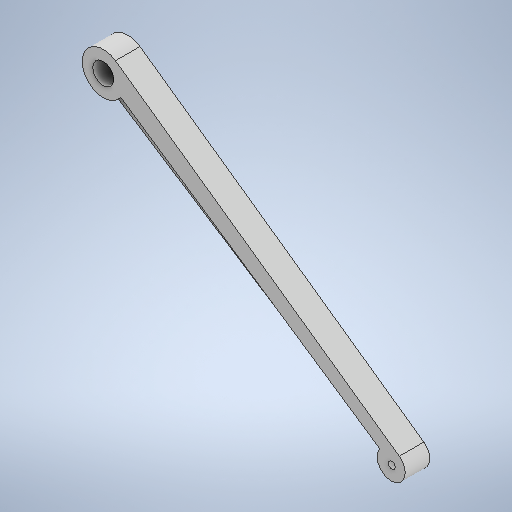
# Autodesk Inventor part: ServoShaft
Saved by Autodesk Inventor 2025.1 (Build 291241000, 241)
## iProperties
Created: 2026-05-06
Part Number: ServoShaft
Material: Generic
Document SubType Name: Modeling
Designer: User
Density: 1 g/cm^3
Appearance: Default
Author: User
## iProperties of the stored document ServoShaft_3DPrint.ipt
Created: 2026-05-06
Part Number: ServoShaft_3DPrint
Material: Generic
Document SubType Name: Modeling
Designer: User
Density: 1 g/cm^3
Appearance: Default
Author: User
Autodesk Inventor part; units mm, degrees
ref_plane "YZ Plane" through (0, 0, 0) normal (1, 0, 0) x (0, 1, 0)
ref_plane "XZ Plane" through (0, 0, 0) normal (0, 1, 0) x (-1, 0, 0)
ref_plane "XY Plane" through (0, 0, 0) normal (0, 0, 1) x (1, 0, 0)
sketch "Sketch1" plane through (0, 0, 0) normal (0, 0, 1) x (1, 0, 0)
  circle A0 centre (9.0361, 0) radius 0.5 projected
  arc A1 (9.1111, -1.9923) -> (9.1111, 1.9923) centre (8.9361, 0) ccw projected
  circle A2 centre (8.9361, 0) radius 2
  point P0 (0, 0)
  point P1 (9.1111, 1.9923)
  point P2 (9.1111, -1.9923)
  constraints: 1 centre point, 1 coincident, 1 concentric
extrude "Extrusion1" add sketch "Sketch1" along normal blind 4
sketch "Sketch2" plane through (8.9361, 0, 0) normal (0, 0, -1) x (-1, 0, 0)
  circle A0 centre (0, 0) radius 2 projected
  circle A1 centre (-0.1, 0) radius 0.5 projected
  point P0 (8.9361, 0)
extrude "Extrusion2" cut sketch "Sketch2" against normal blind 0.5
sketch "Sketch3" plane through (8.9361, 0, 0.5) normal (0, 0, -1) x (-1, 0, 0)
  circle A0 centre (34.6774, 22.9773) radius 1.5 projected
  arc A1 (36.9746, 24.9067) -> (34.2673, 20.0054) centre (34.6774, 22.9773) ccw projected
  circle A2 centre (34.6774, 22.9773) radius 3
  circle A3 centre (41.0489, 27.7862) radius 1.5 projected
  circle A4 centre (41.0489, 27.7862) radius 3
  point P0 (8.9361, 0)
  point P1 (34.2673, 20.0054)
  dimension "d11" = 3
  dimension "d12" = 6
  constraints: 2 centre point, 2 coincident, 1 concentric
  measures "d11" radius of A1
  measures "d12" diameter of A4
extrude "Extrusion3" add sketch "Sketch3" against normal up to surface (3.5 mm away) contours A4
sketch "Sketch6" plane through (8.9361, 0, 0.5) normal (0, 0, -1) x (-1, 0, 0)
  circle A0 centre (41.0489, 27.7862) radius 3 projected
  circle A1 centre (41.0489, 27.7862) radius 1.5 projected
  circle A2 centre (0, 0) radius 2 projected
  circle A3 centre (-0.1, 0) radius 0.5 projected
  line L0 (-1.1543, 1.6333) -> (39.3175, 30.2361)
  line L1 (1.0875, -1.6785) -> (42.6801, 25.2684)
  point P0 (8.9361, 0)
  constraints: 4 end point, 4 point on circle, 4 tangent
extrude "Extrusion6" add sketch "Sketch6" against normal blind 1.75 contours A0 L1 A2 L0
sketch "Sketch7" plane through (8.9361, 0, 2.25) normal (0, 0, 1) x (1, 0, 0)
  line L0 (1.1543, 1.6333) -> (-39.3175, 30.2361) projected
  circle A0 centre (-41.0489, 27.7862) radius 3 projected
  circle A1 centre (0, 0) radius 2 projected
  circle A2 centre (0.1, 0) radius 0.5 projected
  line L1 (0.1, 0) -> (-41.0489, 27.7862)
  point P0 (-8.9361, 0)
  point P1 (-38.5627, 26.1073)
  point P2 (-1.6255, 1.1652)
  constraints: 2 end point, 2 other
extrude "Extrusion7" add sketch "Sketch7" along normal up to surface (1.75 mm away) contours A1 L1 A0 L0
body "Solid1"
